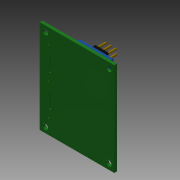
# Autodesk Inventor part: Motherboard_dummy
Saved by Autodesk Inventor 2016 (Build 200138000, 138)
## iProperties
Created: 2014-12-25
Part Number: Motherboard_dummy
Material: ABS Plastic
Document SubType Name: Modeling
Designer: Openlab
Density: 1.06 g/cm^3
Appearance: Smooth - Dark Forest Green
Mass: 9.08054 g
Surface Area: 59.127 cm^2
Volume: 8.56654 cm^3
Author: Openlab
Autodesk Inventor part; units mm, degrees
ref_plane "YZ Plane" through (0, 0, 0) normal (1, 0, 0) x (0, 1, 0)
ref_plane "XZ Plane" through (0, 0, 0) normal (0, 1, 0) x (-1, 0, 0)
ref_plane "XY Plane" through (0, 0, 0) normal (0, 0, 1) x (1, 0, 0)
sketch "Sketch1" plane through (0, 0, 0) normal (0, 1, 0) x (-1, 0, 0)
  line L0 (40, 50) -> (40, 0)
  line L1 (35, 12.25) -> (35, 20.75)
  line L2 (35, 20.75) -> (34, 20.75)
  line L3 (34, 20.75) -> (34, 12.25)
  line L4 (34, 12.25) -> (35, 12.25)
  line L5 (34, 29.25) -> (35, 29.25)
  line L6 (35, 29.25) -> (35, 37.75)
  line L7 (35, 37.75) -> (34, 37.75)
  line L8 (34, 37.75) -> (34, 29.25)
  line L9 (40, 50) -> (0, 50)
  line L10 (0, 0) -> (40, 0)
  line L11 (17.2477, 25) -> (11.4252, 25) construction
  line L12 (0, 0) -> (0, 50)
  circle A0 centre (37, 47) radius 1.5
  circle A1 centre (3, 47) radius 1.5
  circle A2 centre (37, 3) radius 1.5
  circle A3 centre (3, 3) radius 1.5
  point P0 (0, 0)
  point P1 (0, 0)
  point P2 (0, 0)
  point P3 (0, 0)
  point P4 (35.5, 42)
  point P5 (35.5, 25)
  point P6 (35.5, 8)
  dimension "d151" = 8.5
  dimension "d153" = 1
  dimension "d155" = 5
  dimension "d159" = 17
  dimension "d160" = 17
  dimension "d161" = 4.25
  dimension "d162" = 4.25
  dimension "d176" = 4.5
  dimension "d248" = 40
  dimension "d249" = 50
  dimension "d250" = 3
  dimension "d251" = 3
  dimension "d252" = 3
  dimension "d253" = 3
  dimension "d254" = 3
  constraints: 26 end point, 6 perpendicular, 4 centre point, 4 coincident, 4 vertical alignment, 3 equal radius, 2 equal length, 2 horizontal, 2 horizontal alignment, 2 parallel, 2 point on line, 1 collinear, 1 vertical, 1 other
  measures "d151" distance of L7.end L5.start
  measures "d153" distance of L6.end L7.end
  measures "d155" distance between parallel lines of L0 L6
  measures "d159" distance of point (35.5, 25) point (35.5, 42)
  measures "d160" distance of point (35.5, 8) point (35.5, 25)
  measures "d161" distance from line of L7 point (35.5, 42)
  measures "d162" distance from line of point (35.5, 25) L2
  measures "d176" distance from line of L0 point (35.5, 8)
  measures "d248" distance of L0.start L9.end
  measures "d249" distance of L0.start L0.end
  measures "d250" diameter of A0
  measures "d251" distance from line of L0 A0.centre
  measures "d252" distance from line of L9 A0.centre
  measures "d253" distance from line of L10 A3.centre
  measures "d254" distance from line of L12 A3.centre
extrude "Extrusion1" add sketch "Sketch1" against normal blind 1.5
hole "Hole1" at (-35.5, 0, 42) at (-35.5, 0, 25) at (-35.5, 0, 8) direction (0, -1, 0) diameter 1 end through all
sketch "Sketch4" plane through (0, 0, 0) normal (0, 1, 0) x (1, 0, 0)
  line L0 (-7, -46.3) -> (-7, -3)
  line L1 (-7, -3) -> (-25, -3)
  line L2 (-25, -3) -> (-25, -46.3)
  line L3 (-25, -46.3) -> (-7, -46.3)
  line L4 (-40, 0) -> (0, 0) projected
  line L5 (0, 0) -> (0, -50) projected
  dimension "d189" = 18
  dimension "d255" = 3
  dimension "d256" = 7
  dimension "d257" = 43.3
  constraints: 8 end point, 2 vertical, 1 perpendicular
  measures "d189" distance of L0.end L1.end
  measures "d255" distance between parallel lines of L4 L1
  measures "d256" distance between parallel lines of L5 L0
  measures "d257" distance between parallel lines of L3 L1
extrude "Extrusion11" add sketch "Sketch4" along normal blind 5
sketch "Sketch6" plane through (0, 5, 0) normal (0, 1, 0) x (1, 0, 0)
  line L0 (-20.8908, -18.3177) -> (-15.941, -13.368)
  line L1 (-15.941, -13.368) -> (-10.9913, -18.3177)
  line L2 (-10.9913, -18.3177) -> (-15.941, -23.2675)
  line L3 (-15.941, -23.2675) -> (-20.8908, -18.3177)
  point P0 (0, 0)
  dimension "d198" = 7
  dimension "d199" = 7
  constraints: 8 end point, 2 parallel, 1 perpendicular
  measures "d198" distance of L1.end L2.end
  measures "d199" distance of L0.end L1.end
extrude "Extrusion13" add sketch "Sketch6" along normal blind 2
sketch "Sketch7" plane through (0, 5, 0) normal (0, 1, 0) x (1, 0, 0)
  line L0 (-19.1198, -40.3292) -> (-12.1198, -40.3292)
  line L1 (-12.1198, -40.3292) -> (-12.1198, -45.3292)
  line L2 (-12.1198, -45.3292) -> (-19.1198, -45.3292)
  line L3 (-19.1198, -45.3292) -> (-19.1198, -40.3292)
  point P0 (0, 0)
  dimension "d202" = 7
  dimension "d203" = 5
  constraints: 8 end point, 2 parallel, 1 horizontal, 1 perpendicular
  measures "d202" distance of L1.end L2.end
  measures "d203" distance of L2.end L0.start
extrude "Extrusion14" add sketch "Sketch7" along normal blind 2.5
sketch "Sketch8" plane through (0, 7.5, 0) normal (0, 1, 0) x (1, 0, 0)
  line L0 (-18.6618, -41.2282) -> (-17.9618, -41.2282)
  line L1 (-17.9618, -41.2282) -> (-17.9618, -41.9282)
  line L2 (-17.9618, -41.9282) -> (-18.6618, -41.9282)
  line L3 (-18.6618, -41.9282) -> (-18.6618, -41.2282)
  line L4 (-18.6618, -43.9282) -> (-17.9618, -43.9282)
  line L5 (-17.9618, -43.9282) -> (-17.9618, -44.6282)
  line L6 (-17.9618, -44.6282) -> (-18.6618, -44.6282)
  line L7 (-18.6618, -44.6282) -> (-18.6618, -43.9282)
  line L8 (-15.9618, -41.2282) -> (-15.2618, -41.2282)
  line L9 (-15.2618, -41.2282) -> (-15.2618, -41.9282)
  line L10 (-15.2618, -41.9282) -> (-15.9618, -41.9282)
  line L11 (-15.9618, -41.9282) -> (-15.9618, -41.2282)
  line L12 (-15.9618, -43.9282) -> (-15.2618, -43.9282)
  line L13 (-15.2618, -43.9282) -> (-15.2618, -44.6282)
  line L14 (-15.2618, -44.6282) -> (-15.9618, -44.6282)
  line L15 (-15.9618, -44.6282) -> (-15.9618, -43.9282)
  line L16 (-13.2618, -41.2282) -> (-12.5618, -41.2282)
  line L17 (-12.5618, -41.2282) -> (-12.5618, -41.9282)
  line L18 (-12.5618, -41.9282) -> (-13.2618, -41.9282)
  line L19 (-13.2618, -41.9282) -> (-13.2618, -41.2282)
  line L20 (-13.2618, -43.9282) -> (-12.5618, -43.9282)
  line L21 (-12.5618, -43.9282) -> (-12.5618, -44.6282)
  line L22 (-12.5618, -44.6282) -> (-13.2618, -44.6282)
  line L23 (-13.2618, -44.6282) -> (-13.2618, -43.9282)
  point P0 (0, 0)
  dimension "d206" = 0.7
  dimension "d207" = 2
  dimension "d208" = 2
  dimension "d209" = 2
  constraints: 48 end point, 12 parallel, 10 point on line, 6 equal length, 6 horizontal, 6 perpendicular, 2 collinear
  measures "d206" distance of L0.start L0.end
  measures "d207" distance between parallel lines of L4 L2
  measures "d208" distance between parallel lines of L11 L1
  measures "d209" distance between parallel lines of L19 L9
extrude "Extrusion15" add sketch "Sketch8" along normal blind 5
sketch "Sketch9" plane through (-3, 0, 3) normal (0, 0, -1) x (-1, 0, 0)
  line L0 (16.75, 8.5) -> (9.25, 8.5)
  line L1 (9.25, 8.5) -> (9.25, 5)
  line L2 (9.25, 5) -> (16.75, 5)
  line L3 (16.75, 5) -> (16.75, 8.5)
  line L4 (13, 5.7242) -> (13, 7.4058) construction
  line L5 (22, 0) -> (22, 5) projected
  line L6 (4, 5) -> (22, 5) projected
  dimension "d213" = 7.5
  dimension "d214" = 3.5
  dimension "d258" = 5.25
  constraints: 10 end point, 2 parallel, 1 collinear, 1 horizontal, 1 perpendicular, 1 vertical, 1 other
  measures "d213" distance of L0.start L0.end
  measures "d214" distance of L2.end L0.start
  measures "d258" distance between parallel lines of L5 L3
extrude "Extrusion16" add sketch "Sketch9" along normal blind 2 and the other way blind 7
sketch "Sketch15" plane through (-3, 0, 1) normal (0, 0, -1) x (-1, 0, 0)
  line L0 (16.25, 8.25) -> (9.75, 8.25)
  line L1 (9.75, 8.25) -> (9.75, 5.25)
  line L2 (9.75, 5.25) -> (16.25, 5.25)
  line L3 (16.25, 5.25) -> (16.25, 8.25)
  line L4 (9.25, 8.5) -> (9.25, 5) projected
  line L5 (16.75, 8.5) -> (9.25, 8.5) projected
  point P0 (-3, 0)
  dimension "d242" = 6.5
  dimension "d243" = 3
  dimension "d244" = 0.5
  dimension "d245" = 0.25
  constraints: 8 end point, 2 parallel, 1 horizontal, 1 perpendicular
  measures "d242" distance of L0.start L0.end
  measures "d243" distance of L2.end L0.start
  measures "d244" distance between parallel lines of L4 L1
  measures "d245" distance between parallel lines of L0 L5
extrude "Extrusion20" cut sketch "Sketch15" against normal blind 5
body "Solid1"
